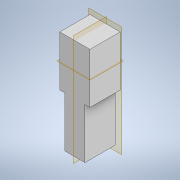
# Autodesk Inventor part: Actuator
Saved by Autodesk Inventor 2021 (Build 250183000, 183)
## iProperties
Created: 2021-03-09
Part Number: Actuator
Material: Generic
Document SubType Name: Modeling
Designer: negt20
Density: 1 g/cm^3
Appearance: Default
Author: negt20
Autodesk Inventor part; units mm, degrees
sketch "Sketch1" plane through (0, 0, 0) normal (0, 0, 1) x (1, 0, 0)
  line L0 (-15, 25) -> (15, 25)
  line L1 (15, 25) -> (15, -25)
  line L2 (15, -25) -> (-15, -25)
  line L3 (-15, -25) -> (-15, 25)
  point P0 (0, 0)
  point P1 (0, 25)
  point P2 (-15, 0)
  dimension "d0" = 50
  dimension "d1" = 30
  constraints: 8 end point, 2 midpoint, 2 parallel, 1 horizontal, 1 horizontal alignment, 1 perpendicular, 1 vertical alignment
  measures "d0" distance of L0.end L1.end
  measures "d1" distance of L0.start L0.end
extrude "Extrusion1" add sketch "Sketch1" along normal blind 30
sketch "Sketch2" plane through (0, 0, 30) normal (0, 0, 1) x (1, 0, 0)
  line L0 (-15, -25) -> (15, -25) projected
  line L1 (-10, -25) -> (10, -25)
  line L2 (10, -25) -> (10, -75)
  line L3 (10, -75) -> (-10, -75)
  line L4 (-10, -75) -> (-10, -25)
  point P0 (0, 0)
  point P1 (0, -25)
  point P2 (0, -25)
  dimension "d4" = 20
  dimension "d5" = 50
  constraints: 8 end point, 2 midpoint, 2 parallel, 1 coincident, 1 horizontal, 1 perpendicular, 1 point on line
  measures "d4" distance of L2.end L3.end
  measures "d5" distance of L1.end L2.end
extrude "Extrusion2" add sketch "Sketch2" against normal blind 30
body "Solid1"
